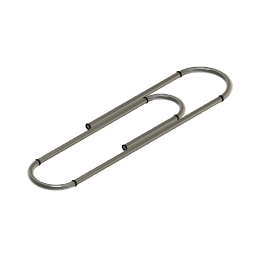
PaperClip (Autodesk Fusion 360 design; units mm, degrees)
part number: 2025-04-19-15-00-37-299
Autodesk Fusion 360 part; units mm, degrees
sketch "Sketch1" plane through (0, 0, 0) normal (0, 0, 1) x (1, 0, 0)
  line L0 (0, 0) -> (0, 26.25)
  line L1 (0, 26.25) -> (-7.5, 26.25) construction
  line L2 (-7.5, 26.25) -> (-7.5, 10)
  line L3 (0, 0) -> (-6.5, 0) construction
  line L4 (-6.5, 0) -> (-6.5, 19.25)
  line L5 (-6.5, 19.25) -> (-1, 19.25) construction
  line L6 (-1, 19.25) -> (-1, 10)
  arc A0 (0, 26.25) -> (-7.5, 26.25) centre (-3.75, 26.25) ccw
  arc A1 (-1, 19.25) -> (-6.5, 19.25) centre (-3.75, 19.25) ccw
  arc A2 (-6.5, 0) -> (0, 0) centre (-3.25, 0) ccw
  dimension "d9" = 26.25
  dimension "d10" = 7.5
  dimension "d11" = 16.25
  dimension "d12" = 6.5
  dimension "d13" = 19.25
  dimension "d14" = 5.5
  dimension "d15" = 9.25
  constraint coincident L0.start L3.start
  constraint vertical L0
  constraint perpendicular L0 L1
  constraint perpendicular L1 L2
  constraint perpendicular L0 L3
  constraint perpendicular L3 L4
  constraint perpendicular L2 L5
  constraint perpendicular L5 L6
  constraint tangent L2 A0
  constraint tangent L4 A1
  measures "d9" distance of L0.start L0.end
  measures "d10" distance of L0.end L1.end
  measures "d11" distance of L1.end L2.end
  measures "d12" distance of L0.start L3.end
  measures "d13" distance of L3.end L4.end
  measures "d14" distance of L4.end L5.end
  measures "d15" distance of L5.end L6.end
sketch "Sketch2" plane through (0, 0, 0) normal (0, 1, 0) x (1, 0, 0)
  circle A0 centre (0, 0) radius 0.375
  dimension "d16" = 0.75
  constraint coincident A0.centre origin
  measures "d16" diameter of A0
sweep "Sweep1" add profiles "Sketch2" path "Sketch1" along L6 A1 L4 A2 L0 A0 L2 section 1
